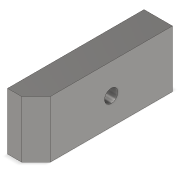
# Autodesk Inventor part: Cover_attachment
Saved by Autodesk Inventor 2020 (Build 240168000, 168)
## iProperties
Created: 2019-05-30
Part Number: Cover_attachment
Material: Steel, Mild
Document SubType Name: Modeling
Designer: chitl
Density: 7.85 g/cm^3
Appearance: Semi-Polished
Author: chitl
Autodesk Inventor part; units mm, degrees
ref_plane "YZ Plane" through (0, 0, 0) normal (1, 0, 0) x (0, 1, 0)
ref_plane "XZ Plane" through (0, 0, 0) normal (0, 1, 0) x (-1, 0, 0)
ref_plane "XY Plane" through (0, 0, 0) normal (0, 0, 1) x (1, 0, 0)
sketch "Sketch1" plane through (0, 0, 0) normal (1, 0, 0) x (0, 1, 0)
  line L0 (6.35, 15.24) -> (-6.35, 15.24)
  line L1 (-6.35, 15.24) -> (-6.35, -15.24)
  line L2 (-6.35, -15.24) -> (6.35, -15.24)
  line L3 (6.35, -15.24) -> (6.35, 15.24)
  line L4 (6.35, 15.24) -> (-6.35, -15.24) construction
  line L5 (-6.35, 15.24) -> (6.35, -15.24) construction
  point P0 (0, 0)
  dimension "d0" = 12.7
  dimension "d1" = 30.48
  constraints: 12 end point, 2 midpoint, 2 parallel, 1 horizontal, 1 perpendicular
  measures "d0" distance of L2.end L1.end
  measures "d1" distance of L1.end L0.end
extrude "Extrusion1" add sketch "Sketch1" along normal blind 6.35
chamfer "Chamfer1" distance 3.175 angle 45 1 edges at (6.35, 0, 15.24)
sketch "Sketch2" plane through (6.35, 0, 0) normal (1, 0, 0) x (0, 0, -1)
  point P0 (0, 0)
  point P1 (1.5638, -0.3192)
hole "Hole1" at (6.35, -0.3192, -1.5638) direction (-1, 0, 0) diameter 3 end through all
body "Solid1"
